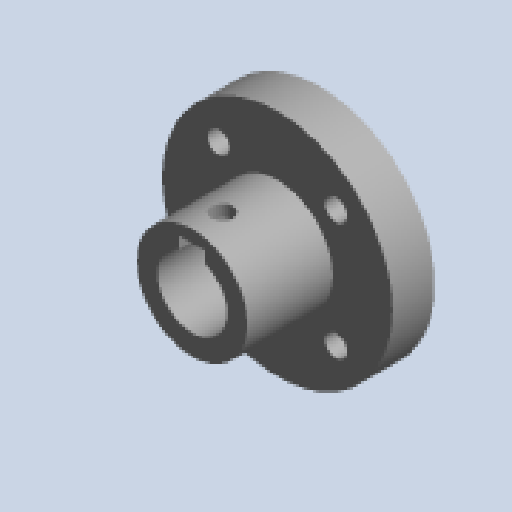
# Autodesk Inventor part: BaseHub
Saved by Autodesk Inventor 2023 (Build 270158000, 158)
## iProperties
Created: 2024-01-25
Part Number: BaseHub
Material: Generic
Document SubType Name: Modeling
Designer: valer
Density: 1 g/cm^3
Appearance: Default
Author: valer
Autodesk Inventor part; units mm, degrees
ref_plane "YZ Plane" through (0, 0, 0) normal (1, 0, 0) x (0, 1, 0)
ref_plane "XZ Plane" through (0, 0, 0) normal (0, 1, 0) x (-1, 0, 0)
ref_plane "XY Plane" through (0, 0, 0) normal (0, 0, 1) x (1, 0, 0)
sketch "Hub" plane through (0, 0, 0) normal (0, 0, 1) x (1, 0, 0)
  circle A0 centre (0, 0) radius 6.6 construction
  circle A1 centre (-6.9148, 6.9148) radius 1.5875 construction
  circle A2 centre (6.9148, 6.9148) radius 1.5875 construction
  circle A3 centre (-6.9148, -6.9148) radius 1.5875 construction
  circle A4 centre (6.9148, -6.9148) radius 1.5875 construction
  line L0 (-6.9148, 6.9148) -> (6.9148, 6.9148) construction
  line L1 (6.9148, 6.9148) -> (6.9148, -6.9148) construction
  line L2 (6.9148, -6.9148) -> (-6.9148, -6.9148) construction
  line L3 (-6.9148, -6.9148) -> (-6.9148, 6.9148) construction
  circle A5 centre (0, 0) radius 12.958 construction
  line L4 (-6.9148, -6.9148) -> (6.9148, 6.9148) construction
  line L5 (-6.9148, 6.9148) -> (-5.7923, 5.7923) construction
  line L6 (-5.7923, 5.7923) -> (-4.6669, 4.6669) construction
  line L7 (-8.0373, 8.0373) -> (-9.1627, 9.1627) construction
  circle A6 centre (0, 0) radius 4
  line L8 (0, 4) -> (0, 5.05) construction
  line L9 (0, -21.8312) -> (0, 19.0969) construction
  line L10 (-1.475, 5.05) -> (1.475, 5.05)
  line L11 (-1.475, 5.05) -> (-1.475, 3.7181)
  line L12 (1.475, 5.05) -> (1.475, 3.7181)
  circle A7 centre (0, 0) radius 13.25
  circle A8 centre (6.9148, 6.9148) radius 1.2891
  circle A9 centre (6.9148, -6.9148) radius 1.2891
  circle A10 centre (-6.9148, -6.9148) radius 1.2891
  circle A11 centre (-6.9148, 6.9148) radius 1.2891
  circle A12 centre (6.9148, -6.9148) radius 2.84 construction
  circle A13 centre (12.3744, -12.3744) radius 1.621 construction
  circle A14 centre (12.3744, -12.3744) radius 3.61 construction
  dimension "d0" = 13.2
  dimension "d1" = 3.175
  dimension "d5" = 13.8296
  dimension "d6" = 45
  dimension "d9" = 8
  dimension "d10" = 1.05
  dimension "d11" = 2.95
  dimension "d21" = 2.5781
  dimension "d27" = 26.5
  dimension "d34" = 5.68
  dimension "d35" = 7.22
  constraints: 24 end point, 15 coincident, 12 centre point, 6 equal radius, 5 point on circle, 3 collinear, 3 vertical, 2 equal length, 2 horizontal, 2 midpoint, 2 parallel, 1 perpendicular, 6 other
  measures "d1" diameter of A1
  measures "d5" distance of L0.start L0.end
  measures "d6" angle of L0 L5
  measures "d9" diameter of A6
  measures "d10" distance of L8.end L8.start
  measures "d11" distance of L10.start L10.end
  measures "d21" diameter of A8
  measures "d27" diameter of A7
  measures "d34" diameter of A12
  measures "d35" diameter of A14
extrude "HubFeature" add sketch "Hub" against normal blind 5
sketch "Lip" plane through (0, 0, 0) normal (0, 0, 1) x (1, 0, 0)
  circle A0 centre (0, 0) radius 6.5
  line L0 (-1.5, 5.075) -> (1.5, 5.075)
  line L1 (-1.5, 3.7351) -> (-1.5, 5.075)
  line L2 (1.5, 5.075) -> (1.5, 3.7351)
  arc A1 (-1.5, 3.7351) -> (1.5, 3.7351) centre (0, 0) ccw
  line L3 (0, 0) -> (0, 5.075) construction
  line L4 (-1.475, 5.05) -> (1.475, 5.05) projected
  line L5 (-1.475, 3.7181) -> (-1.475, 5.05) projected
  dimension "d28" = 13
  dimension "d29" = 4.025
  dimension "d36" = 0.025
  dimension "d37" = 0.025
  constraints: 8 end point, 3 perpendicular, 2 centre point, 2 point on circle, 1 coincident, 1 concentric, 1 horizontal, 1 midpoint
  measures "d28" diameter of A0
  measures "d29" radius of A1
  measures "d36" distance between parallel lines of L0 L4
  measures "d37" distance between parallel lines of L1 L5
extrude "LipFeature" add sketch "Lip" along normal blind 10
sketch "Sketch6" plane through (0, 0, 0) normal (0, 1, 0) x (-1, 0, 0)
  line L0 (6.5, 10) -> (-6.5, 10) construction
  line L1 (0, 10) -> (0, 0) construction
  circle A0 centre (0, 6.5) radius 1.25
  dimension "d30" = 2.5
  dimension "d31" = 3.5
  constraints: 2 end point, 1 centre point, 1 midpoint, 1 point on line, 1 vertical
  measures "d30" diameter of A0
  measures "d31" distance from line of L0 A0.centre
extrude "Extrusion5" cut sketch "Sketch6" along normal blind 10
body "Solid1"
